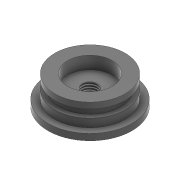
# Autodesk Inventor part: Pieza_sonar
Saved by Autodesk Inventor 2022.3 (Build 263350000, 350)
## iProperties
Created: 2023-07-17
Part Number: Pieza_sonar
Material: Genérico
Document SubType Name: Modeling
Designer: Usuario
Density: 1 g/cm^3
Appearance: Valor por defecto
Author: Usuario
Autodesk Inventor part; units mm, degrees
ref_plane "YZ Plane" through (0, 0, 0) normal (1, 0, 0) x (0, 1, 0)
ref_plane "XZ Plane" through (0, 0, 0) normal (0, 1, 0) x (-1, 0, 0)
sketch "Boceto1" plane through (0, 0, 0) normal (0, 1, 0) x (-1, 0, 0)
  circle A0 centre (0, 0) radius 26
  dimension "d0" = 52
  constraints: 1 centre point, 1 coincident
  measures "d0" diameter of A0
extrude "Extrusión1" add sketch "Boceto1" along normal blind 4
sketch "Boceto2" plane through (0, 4, 0) normal (0, 1, 0) x (1, 0, 0)
  circle A0 centre (0, 0) radius 21.775
  dimension "d3" = 43.55
  constraints: 1 centre point, 1 coincident
  measures "d3" diameter of A0
extrude "Extrusión2" add sketch "Boceto2" along normal blind 13.8
sketch "Boceto3" plane through (0, 17.8, 0) normal (0, 1, 0) x (1, 0, 0)
  circle A0 centre (0, 0) radius 13.875
  dimension "d6" = 27.75
  constraints: 1 centre point, 1 coincident
  measures "d6" diameter of A0
extrude "Extrusión3" cut sketch "Boceto3" against normal blind 7.85
sketch "Boceto4" plane through (0, 9.95, 0) normal (0, 1, 0) x (1, 0, 0)
  circle A0 centre (0, 0) radius 4.8
  dimension "d9" = 9.6
  constraints: 1 centre point, 1 coincident
  measures "d9" diameter of A0
extrude "Extrusión4" cut sketch "Boceto4" against normal blind 12
sketch "Boceto5" plane through (0, 0, 0) normal (0, -1, 0) x (1, 0, 0)
  circle A0 centre (0, 0) radius 21.2
  dimension "d12" = 42.4
  constraints: 1 centre point, 1 coincident
  measures "d12" diameter of A0
extrude "Extrusión5" cut sketch "Boceto5" against normal blind 3
thread "Rosca1" size "M10x1.5" class "6H" standard "ANSI Metric M Profile" full length
ref_plane "Plano de trabajo1" through (0, 14.2, 0) normal (0, 1, 0) x (1, 0, 0)
sketch "Boceto6" plane through (0, 14.2, 0) normal (0, 1, 0) x (1, 0, 0)
  circle A0 centre (0, 0) radius 21.775
  circle A1 centre (0, 0) radius 18.925
  dimension "d18" = 37.85
  constraints: 2 centre point, 2 coincident
  measures "d18" diameter of A1
extrude "Extrusión6" cut sketch "Boceto6" against normal blind 5
